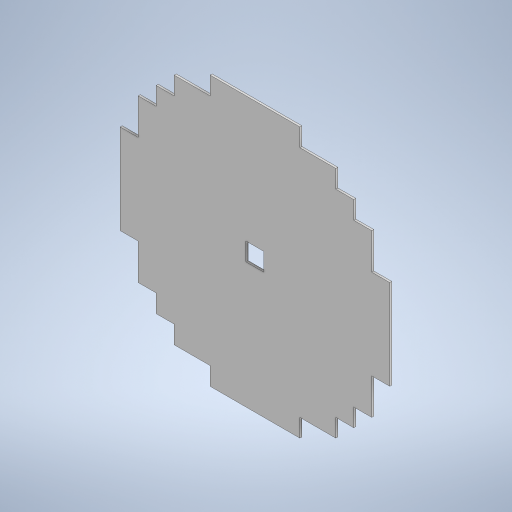
# Autodesk Inventor part: Disc 4
Saved by Autodesk Inventor 2024 (Build 280153000, 153)
## iProperties
Created: 2024-02-02
Part Number: Disc 4
Material: Generic
Document SubType Name: Modeling
Designer: newic
Density: 1 g/cm^3
Appearance: Default
Author: newic
Autodesk Inventor part; units mm, degrees
ref_plane "YZ Plane" through (0, 0, 0) normal (1, 0, 0) x (0, 1, 0)
ref_plane "XZ Plane" through (0, 0, 0) normal (0, 1, 0) x (-1, 0, 0)
ref_plane "XY Plane" through (0, 0, 0) normal (0, 0, 1) x (1, 0, 0)
sketch "Sketch1" plane through (0, 0, 0) normal (0, 0, 1) x (1, 0, 0)
  circle A0 centre (0, 0) radius 152.4
  circle A1 centre (0, 0) radius 5.5
  dimension "d0" = 304.8
  dimension "d1" = 11
  constraints: 2 centre point, 2 coincident
  measures "d0" diameter of A0
  measures "d1" diameter of A1
extrude "Extrusion1" add sketch "Sketch1" along normal blind 2.2
fillet "Fillet1" radius 1.1 2 edges at (-152.4, 0, 0) (-152.4, 0, 2.2)
sketch "Sketch2" plane through (0, 0, 2.2) normal (0, 0, 1) x (1, 0, 0)
  line L0 (206.2137, 42.4617) -> (289.822, 42.4617) construction
  line L1 (289.822, 42.4617) -> (289.822, -13.3654) construction
  line L2 (289.822, -13.3654) -> (206.2137, -13.3654) construction
  line L3 (206.2137, -13.3654) -> (206.2137, 42.4617) construction
  line L4 (9.525, 9.525) -> (-9.525, 9.525)
  line L5 (-9.525, 9.525) -> (-9.525, -9.525)
  line L6 (-9.525, -9.525) -> (9.525, -9.525)
  line L7 (9.525, -9.525) -> (9.525, 9.525)
  line L8 (-123.825, 47.625) -> (-104.775, 47.625)
  line L9 (-123.825, -47.625) -> (-142.875, -47.625)
  line L10 (-123.825, -47.625) -> (-104.775, -47.625)
  line L11 (0, 9.525) -> (0, -9.525)
  line L12 (-9.525, 0) -> (9.525, 0)
  line L13 (0, 0) -> (-4.1012, 3.8959)
  line L14 (-142.875, 28.575) -> (-123.825, 28.575)
  line L15 (-123.825, 28.575) -> (-123.825, 9.525)
  line L16 (-123.825, 9.525) -> (-142.875, 9.525)
  line L17 (-142.875, 9.525) -> (-142.875, 28.575)
  line L18 (-142.875, -9.525) -> (-123.825, -9.525)
  line L19 (-123.825, -9.525) -> (-123.825, 9.525)
  line L20 (-142.875, 9.525) -> (-142.875, -9.525)
  line L21 (-123.825, -47.625) -> (-123.825, -28.575)
  line L22 (-123.825, -28.575) -> (-142.875, -28.575)
  line L23 (-142.875, -28.575) -> (-142.875, -47.625)
  line L24 (-123.825, -9.525) -> (-123.825, -28.575)
  line L25 (-142.875, -28.575) -> (-142.875, -9.525)
  line L26 (-123.825, 47.625) -> (-104.775, 47.625)
  line L27 (-104.775, 47.625) -> (-104.775, 66.675)
  line L28 (-104.775, 66.675) -> (-123.825, 66.675)
  line L29 (-123.825, 66.675) -> (-123.825, 47.625)
  line L30 (-123.825, -47.625) -> (-104.775, -47.625)
  line L31 (-104.775, -47.625) -> (-104.775, -66.675)
  line L32 (-104.775, -66.675) -> (-123.825, -66.675)
  line L33 (-123.825, -66.675) -> (-123.825, -47.625)
  circle A0 centre (0, 0) radius 350.7035
  line L34 (-123.825, -85.725) -> (-104.775, -85.725)
  line L35 (-123.825, -85.725) -> (-104.775, -85.725)
  line L36 (-104.775, -85.725) -> (-104.775, -66.675)
  line L37 (-123.825, -66.675) -> (-123.825, -85.725)
  line L38 (-123.825, 85.725) -> (-104.775, 85.725)
  line L39 (-123.825, 85.725) -> (-104.775, 85.725)
  line L40 (-104.775, 85.725) -> (-104.775, 66.675)
  line L41 (-123.825, 66.675) -> (-123.825, 85.725)
  line L42 (-104.775, 85.725) -> (-85.725, 85.725)
  line L43 (-85.725, 85.725) -> (-85.725, 104.775)
  line L44 (-85.725, 104.775) -> (-104.775, 104.775)
  line L45 (-104.775, 104.775) -> (-104.775, 85.725)
  line L46 (-104.775, -85.725) -> (-85.725, -85.725)
  line L47 (-85.725, -85.725) -> (-85.725, -104.775)
  line L48 (-85.725, -104.775) -> (-104.775, -104.775)
  line L49 (-104.775, -104.775) -> (-104.775, -85.725)
  line L50 (-85.725, 104.775) -> (-66.675, 104.775)
  line L51 (-66.675, 104.775) -> (-66.675, 123.825)
  line L52 (-66.675, 123.825) -> (-85.725, 123.825)
  line L53 (-85.725, 123.825) -> (-85.725, 104.775)
  line L54 (-85.725, -104.775) -> (-66.675, -104.775)
  line L55 (-66.675, -104.775) -> (-66.675, -123.825)
  line L56 (-66.675, -123.825) -> (-85.725, -123.825)
  line L57 (-85.725, -123.825) -> (-85.725, -104.775)
  line L58 (-142.875, 28.575) -> (-123.825, 28.575)
  line L59 (-123.825, 28.575) -> (-123.825, 47.625)
  line L60 (-123.825, 47.625) -> (-142.875, 47.625)
  line L61 (-142.875, 47.625) -> (-142.875, 28.575)
  line L62 (-47.625, 104.775) -> (-66.675, 104.775)
  line L63 (-66.675, 123.825) -> (-47.625, 123.825)
  line L64 (-47.625, 123.825) -> (-47.625, 104.775)
  line L65 (-47.625, -104.775) -> (-66.675, -104.775)
  line L66 (-66.675, -123.825) -> (-47.625, -123.825)
  line L67 (-47.625, -123.825) -> (-47.625, -104.775)
  line L68 (-47.625, 123.825) -> (-28.575, 123.825)
  line L69 (-28.575, 123.825) -> (-28.575, 142.875)
  line L70 (-28.575, 142.875) -> (-47.625, 142.875)
  line L71 (-47.625, 142.875) -> (-47.625, 123.825)
  line L72 (-47.625, -123.825) -> (-28.575, -123.825)
  line L73 (-28.575, -123.825) -> (-28.575, -142.875)
  line L74 (-28.575, -142.875) -> (-47.625, -142.875)
  line L75 (-47.625, -142.875) -> (-47.625, -123.825)
  line L76 (-9.525, 123.825) -> (-28.575, 123.825)
  line L77 (-28.575, 142.875) -> (-9.525, 142.875)
  line L78 (-9.525, 142.875) -> (-9.525, 123.825)
  line L79 (-9.525, -123.825) -> (-28.575, -123.825)
  line L80 (-28.575, -142.875) -> (-9.525, -142.875)
  line L81 (-9.525, -142.875) -> (-9.525, -123.825)
  line L82 (9.525, 123.825) -> (9.525, 142.875)
  line L83 (9.525, -123.825) -> (9.525, -142.875)
  line L84 (-9.525, 123.825) -> (9.525, 123.825)
  line L85 (9.525, 142.875) -> (-9.525, 142.875)
  line L86 (-9.525, -123.825) -> (9.525, -123.825)
  line L87 (9.525, -142.875) -> (-9.525, -142.875)
  line L88 (9.525, 9.525) -> (9.525, -9.525)
  line L89 (-9.525, 9.525) -> (9.525, 9.525)
  line L90 (9.525, -9.525) -> (-9.525, -9.525)
  line L91 (-9.525, -9.525) -> (-9.525, 9.525)
  line L92 (123.825, 47.625) -> (104.775, 47.625)
  line L93 (123.825, -47.625) -> (104.775, -47.625)
  line L94 (123.825, -47.625) -> (142.875, -47.625)
  line L95 (9.525, 0) -> (-9.525, 0)
  line L96 (0, 0) -> (4.1012, 3.8959)
  line L97 (142.875, 28.575) -> (123.825, 28.575)
  line L98 (123.825, 28.575) -> (123.825, 9.525)
  line L99 (123.825, 9.525) -> (142.875, 9.525)
  line L100 (142.875, 9.525) -> (142.875, 28.575)
  line L101 (123.825, -9.525) -> (123.825, 9.525)
  line L102 (142.875, -9.525) -> (123.825, -9.525)
  line L103 (142.875, 9.525) -> (142.875, -9.525)
  line L104 (123.825, -9.525) -> (123.825, -28.575)
  line L105 (123.825, -47.625) -> (123.825, -28.575)
  line L106 (142.875, -28.575) -> (142.875, -9.525)
  line L107 (123.825, -28.575) -> (142.875, -28.575)
  line L108 (142.875, -28.575) -> (142.875, -47.625)
  line L109 (123.825, 47.625) -> (104.775, 47.625)
  line L110 (104.775, 47.625) -> (104.775, 66.675)
  line L111 (104.775, 66.675) -> (123.825, 66.675)
  line L112 (123.825, 66.675) -> (123.825, 47.625)
  line L113 (123.825, -47.625) -> (104.775, -47.625)
  line L114 (104.775, -47.625) -> (104.775, -66.675)
  line L115 (104.775, -66.675) -> (123.825, -66.675)
  line L116 (123.825, -66.675) -> (123.825, -47.625)
  line L117 (123.825, -85.725) -> (104.775, -85.725)
  line L118 (104.775, -85.725) -> (104.775, -66.675)
  line L119 (123.825, -66.675) -> (123.825, -85.725)
  line L120 (123.825, -85.725) -> (104.775, -85.725)
  line L121 (123.825, 85.725) -> (104.775, 85.725)
  line L122 (104.775, 85.725) -> (104.775, 66.675)
  line L123 (123.825, 85.725) -> (104.775, 85.725)
  line L124 (123.825, 66.675) -> (123.825, 85.725)
  line L125 (104.775, 85.725) -> (85.725, 85.725)
  line L126 (85.725, 85.725) -> (85.725, 104.775)
  line L127 (85.725, 104.775) -> (104.775, 104.775)
  line L128 (104.775, 104.775) -> (104.775, 85.725)
  line L129 (104.775, -85.725) -> (85.725, -85.725)
  line L130 (85.725, -85.725) -> (85.725, -104.775)
  line L131 (85.725, -104.775) -> (104.775, -104.775)
  line L132 (104.775, -104.775) -> (104.775, -85.725)
  line L133 (85.725, 104.775) -> (66.675, 104.775)
  line L134 (66.675, 104.775) -> (66.675, 123.825)
  line L135 (66.675, 123.825) -> (85.725, 123.825)
  line L136 (85.725, 123.825) -> (85.725, 104.775)
  line L137 (85.725, -104.775) -> (66.675, -104.775)
  line L138 (66.675, -104.775) -> (66.675, -123.825)
  line L139 (66.675, -123.825) -> (85.725, -123.825)
  line L140 (85.725, -123.825) -> (85.725, -104.775)
  line L141 (142.875, 28.575) -> (123.825, 28.575)
  line L142 (123.825, 28.575) -> (123.825, 47.625)
  line L143 (123.825, 47.625) -> (142.875, 47.625)
  line L144 (142.875, 47.625) -> (142.875, 28.575)
  line L145 (47.625, 104.775) -> (66.675, 104.775)
  line L146 (66.675, 123.825) -> (47.625, 123.825)
  line L147 (47.625, 123.825) -> (47.625, 104.775)
  line L148 (47.625, -104.775) -> (66.675, -104.775)
  line L149 (47.625, -123.825) -> (47.625, -104.775)
  line L150 (66.675, -123.825) -> (47.625, -123.825)
  line L151 (47.625, 123.825) -> (28.575, 123.825)
  line L152 (28.575, 123.825) -> (28.575, 142.875)
  line L153 (28.575, 142.875) -> (47.625, 142.875)
  line L154 (47.625, 142.875) -> (47.625, 123.825)
  line L155 (47.625, -123.825) -> (28.575, -123.825)
  line L156 (28.575, -123.825) -> (28.575, -142.875)
  line L157 (28.575, -142.875) -> (47.625, -142.875)
  line L158 (47.625, -142.875) -> (47.625, -123.825)
  line L159 (9.525, 123.825) -> (28.575, 123.825)
  line L160 (9.525, 142.875) -> (9.525, 123.825)
  line L161 (28.575, 142.875) -> (9.525, 142.875)
  line L162 (9.525, -142.875) -> (9.525, -123.825)
  line L163 (9.525, -123.825) -> (28.575, -123.825)
  line L164 (28.575, -142.875) -> (9.525, -142.875)
  line L165 (-9.525, 123.825) -> (-9.525, 142.875)
  line L166 (9.525, 123.825) -> (-9.525, 123.825)
  line L167 (-9.525, 142.875) -> (9.525, 142.875)
  line L168 (-9.525, -123.825) -> (-9.525, -142.875)
  line L169 (9.525, -123.825) -> (-9.525, -123.825)
  line L170 (-9.525, -142.875) -> (9.525, -142.875)
  point P0 (-123.825, -9.525)
  point P1 (-123.825, -47.625)
  point P2 (-123.825, -85.725)
  point P3 (123.825, -9.525)
  point P4 (123.825, -47.625)
  point P5 (123.825, -85.725)
  dimension "d22" = 19.05
  dimension "d23" = 19.05
  dimension "d29" = 19.05
  dimension "d30" = 19.05
  dimension "d35" = 19.05
  dimension "d36" = 19.05
  dimension "d67" = 19.05
  dimension "d68" = 19.05
  dimension "d69" = 19.05
  dimension "d70" = 19.05
  dimension "d71" = 19.05
  dimension "d72" = 19.05
  dimension "d73" = 19.05
  dimension "d74" = 19.05
  dimension "d77" = 19.05
  dimension "d78" = 19.05
  dimension "d79" = 19.05
  dimension "d80" = 19.05
  constraints: 334 end point, 98 symmetric about line, 20 parallel, 10 horizontal, 10 perpendicular, 5 midpoint, 2 coincident, 1 centre point, 2 other
  measures "d22" distance of L15.end L16.end
  measures "d23" distance of L15.start L15.end
  measures "d29" distance of L28.end L27.end
  measures "d30" distance of L27.end L26.end
  measures "d35" distance of L31.end L32.end
  measures "d36" distance of L30.end L31.end
  measures "d67" distance of L44.end L43.end
  measures "d68" distance of L43.end L42.end
  measures "d69" distance of L47.end L48.end
  measures "d70" distance of L46.end L47.end
  measures "d71" distance of L52.end L51.end
  measures "d72" distance of L51.end L50.end
  measures "d73" distance of L55.end L56.end
  measures "d74" distance of L54.end L55.end
  measures "d77" distance of L70.end L69.end
  measures "d78" distance of L69.end L68.end
  measures "d79" distance of L73.end L74.end
  measures "d80" distance of L72.end L73.end
extrude "Extrusion2" cut sketch "Sketch2" against normal blind 25.4
body "Solid1"
